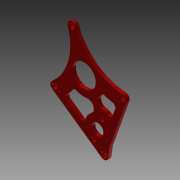
# Autodesk Inventor part: OutlineSketch1
Saved by Autodesk Inventor 2013 (Build 170138000, 138)
## iProperties
Created: 2013-06-03
Part Number: OutlineSketch1
Material: Aluminum 6061
Document SubType Name: Modeling
Designer: mvarma
Density: 2.71 g/cm^3
Author: mvarma
Autodesk Inventor part; units mm, degrees
ref_plane "YZ Plane" through (0, 0, 0) normal (1, 0, 0) x (0, 1, 0)
ref_plane "XZ Plane" through (0, 0, 0) normal (0, 1, 0) x (-1, 0, 0)
ref_plane "XY Plane" through (0, 0, 0) normal (0, 0, 1) x (1, 0, 0)
sketch "Sketch1" plane through (0, 0, 0) normal (0, 0, 1) x (1, 0, 0)
  line L0 (0, 0) -> (304.8, 0) construction
  line L1 (304.8, 0) -> (304.8, 50.8) construction
  line L2 (304.8, 50.8) -> (0, 50.8) construction
  line L3 (0, 50.8) -> (0, 0) construction
  circle A0 centre (152.4, 23.8125) radius 6.35 construction
  circle A1 centre (152.4, 23.8125) radius 34.29 construction
  circle A2 centre (152.4, 23.8125) radius 22.225 construction
  line L4 (152.4, 23.8125) -> (139.52, 61.741) construction
  circle A3 centre (139.52, 61.741) radius 9.525 construction
  circle A4 centre (139.52, 61.741) radius 17.78 construction
  circle A5 centre (91.5619, 85.09) radius 31.75 construction
  circle A6 centre (163.3424, 109.4657) radius 31.75 construction
  circle A7 centre (222.6465, 85.09) radius 31.75 construction
  line L5 (0, 50.8) -> (0, 53.34) construction
  line L6 (0, 53.34) -> (304.8, 53.34) construction
  line L7 (304.8, 53.34) -> (304.8, 50.8) construction
  circle A8 centre (139.52, 61.741) radius 21.59 construction
  circle A9 centre (152.4, 23.8125) radius 46.99 construction
  circle A10 centre (152.4, 23.8125) radius 50.8 construction
  arc A11 (86.3865, 79.4564) -> (92.4363, 92.6899) centre (91.5619, 85.09) ccw construction
  circle A12 centre (163.3424, 109.4657) radius 7.65 construction
  arc A13 (222.2546, 92.73) -> (226.29, 78.3634) centre (222.6465, 85.09) ccw construction
  circle A14 centre (163.3424, 109.4657) radius 9.1 construction
  circle A15 centre (139.52, 61.741) radius 22.9 construction
  line L8 (86.3865, 79.4564) -> (124.0276, 44.8769) construction
  line L9 (170.8782, 108.1486) -> (162.078, 57.7984) construction
  line L10 (92.4363, 92.6899) -> (91.5619, 85.09) construction
  line L11 (91.5619, 85.09) -> (86.3865, 79.4564) construction
  arc A16 (128.9499, 92.8673) -> (131.407, 97.9722) centre (127.6738, 96.6252) ccw
  circle A17 centre (127.6738, 96.6252) radius 7.9375 construction
  line L12 (92.4363, 92.6899) -> (126.7664, 88.7398) construction
  line L13 (133.1953, 90.9229) -> (158.0208, 114.9615) construction
  line L14 (158.0208, 114.9615) -> (163.3424, 109.4657) construction
  line L15 (170.8782, 108.1486) -> (163.3424, 109.4657) construction
  line L16 (139.52, 61.741) -> (127.6738, 96.6252) construction
  line L17 (91.5619, 85.09) -> (163.3424, 109.4657) construction
  line L18 (152.4, 23.8125) -> (91.5619, 85.09) construction
  line L19 (152.4, 23.8125) -> (163.3424, 109.4657) construction
  circle A18 centre (127.6738, 96.6252) radius 9.2075 construction
  circle A19 centre (127.6738, 96.6252) radius 6.1595 construction
  arc A20 (92.4363, 92.6899) -> (86.3865, 79.4564) centre (91.5619, 85.09) ccw construction
  circle A21 centre (163.3424, 109.4657) radius 25.4 construction
  circle A22 centre (222.6465, 85.09) radius 25.4 construction
  line L20 (104.7627, 113.9656) -> (78.361, 56.2144) construction
  circle A23 centre (91.5619, 85.09) radius 25.4 construction
  line L21 (214.0607, 115.6571) -> (231.2324, 54.5229) construction
  line L22 (56.0019, 185.6657) -> (208.4019, 185.6657)
  line L23 (208.4019, 185.6657) -> (208.4019, -4.8343)
  line L24 (208.4019, -4.8343) -> (56.0019, -4.8343)
  line L25 (56.0019, -4.8343) -> (56.0019, 185.6657)
  circle A24 centre (139.52, 61.741) radius 11.1125
  arc A25 (226.1312, 75.4959) -> (221.6192, 95.3086) centre (223.8752, 85.4023) ccw construction
  line L26 (221.4349, 84.7168) -> (229.5152, 60.6363) construction
  line L27 (223.8752, 85.4023) -> (229.5152, 60.6363) construction
  line L28 (221.4349, 84.7168) -> (213.3547, 108.7973) construction
  line L29 (223.8752, 85.4023) -> (218.2352, 110.1682) construction
  arc A26 (212.5972, 111.0549) -> (214.1122, 106.5398) centre (213.3547, 108.7973) ccw construction
  arc A27 (218.764, 107.8464) -> (217.7065, 112.49) centre (218.2352, 110.1682) ccw construction
  arc A28 (218.764, 107.8464) -> (214.1122, 106.5398) centre (229.5152, 60.6363) ccw construction
  arc A29 (217.7065, 112.49) -> (212.5972, 111.0549) centre (229.5152, 60.6363) ccw construction
  line L30 (213.3547, 108.7973) -> (212.5972, 111.0549) construction
  line L31 (218.2352, 110.1682) -> (217.7065, 112.49) construction
  arc A30 (221.6192, 95.3086) -> (218.2029, 94.349) centre (229.5152, 60.6363) ccw construction
  arc A31 (226.1312, 75.4959) -> (224.667, 75.0846) centre (229.5152, 60.6363) ccw construction
  line L32 (104.4015, 107.0791) -> (92.7013, 84.5343) construction
  line L33 (81.0012, 61.9895) -> (90.3961, 85.5882) construction
  arc A32 (100.6718, 111.3992) -> (98.9102, 106.9744) centre (99.791, 109.1868) ccw construction
  arc A33 (103.3046, 104.9655) -> (105.4983, 109.1926) centre (104.4015, 107.0791) ccw construction
  arc A34 (103.3046, 104.9655) -> (98.9102, 106.9744) centre (81.0012, 61.9895) ccw construction
  line L34 (99.791, 109.1868) -> (100.6718, 111.3992) construction
  line L35 (104.4015, 107.0791) -> (105.4983, 109.1926) construction
  arc A35 (105.4983, 109.1926) -> (100.6718, 111.3992) centre (81.0012, 61.9895) ccw construction
  arc A36 (218.2029, 94.349) -> (224.667, 75.0846) centre (221.4349, 84.7168) ccw construction
  arc A37 (88.0213, 75.5164) -> (97.3814, 93.5522) centre (92.7013, 84.5343) ccw construction
  line L36 (90.3961, 85.5882) -> (99.791, 109.1868) construction
  line L37 (92.7013, 84.5343) -> (81.0012, 61.9895) construction
  arc A38 (88.0213, 75.5164) -> (86.6381, 76.1487) centre (81.0012, 61.9895) ccw construction
  arc A39 (97.3814, 93.5522) -> (94.1541, 95.0276) centre (81.0012, 61.9895) ccw construction
  arc A40 (94.1541, 95.0276) -> (86.6381, 76.1487) centre (90.3961, 85.5882) ccw construction
  line L38 (163.3424, 109.4657) -> (140.8985, 121.3583) construction
  line L39 (163.3424, 109.4657) -> (185.7862, 97.5731) construction
  circle A41 centre (139.52, 61.741) radius 26.71 construction
  line L40 (222.2546, 92.73) -> (138.1517, 88.4159) construction
  line L41 (226.29, 78.3634) -> (152.2412, 38.2549) construction
  line L42 (222.6465, 85.09) -> (222.2546, 92.73) construction
  line L43 (222.6465, 85.09) -> (226.29, 78.3634) construction
  line L44 (139.52, 61.741) -> (138.1517, 88.4159) construction
  line L45 (139.52, 61.741) -> (152.2412, 38.2549) construction
  arc A42 (226.29, 78.3634) -> (222.2546, 92.73) centre (222.6465, 85.09) ccw construction
  arc A43 (226.29, 78.3634) -> (225.5574, 78.0155) centre (222.6465, 85.09) ccw construction
  line L46 (139.52, 61.741) -> (222.6465, 85.09) construction
  circle A44 centre (139.52, 61.741) radius 15.875
  arc A45 (108.721, 42.0202) -> (123.8923, 95.4203) centre (76.0203, 80.1659) ccw
  arc A46 (131.407, 97.9722) -> (175.959, 64.8533) centre (178.6686, 115.0239) ccw
  circle A47 centre (152.4, 23.8125) radius 11.176 construction
  line L47 (152.4, 23.8125) -> (158.5256, 5.7742) construction
  circle A48 centre (152.4, 23.8125) radius 5.5065
  line L48 (156.5338, 34.1959) -> (148.2662, 13.4291) construction
  circle A49 centre (156.5338, 34.1959) radius 2.1082
  circle A50 centre (148.2662, 13.4291) radius 2.1082
  arc A51 (166.3874, 21.8643) -> (163.8992, 15.6142) centre (152.4, 23.8125) ccw
  circle A52 centre (111.304, 39.007) radius 9.525 construction
  circle A53 centre (175.745, 60.8903) radius 9.525 construction
  arc A54 (109.2416, 42.3978) -> (109.0199, 35.7614) centre (111.304, 39.007) ccw
  arc A55 (179.4939, 59.5878) -> (175.3161, 64.8358) centre (175.745, 60.8903) ccw
  arc A56 (157.2494, 9.5322) -> (156.2414, 2.5286) centre (158.5256, 5.7742) ccw
  line L49 (152.4, 23.8125) -> (165.1433, 18.7393) construction
  line L50 (166.3874, 21.8643) -> (163.8992, 15.6142)
  arc A57 (163.8992, 15.6142) -> (166.3874, 21.8643) centre (152.4, 23.8125) ccw construction
  line L51 (163.8992, 15.6142) -> (162.4566, 5.2282)
  line L52 (156.2414, 2.5286) -> (109.0199, 35.7614)
  line L53 (166.3874, 21.8643) -> (179.4939, 59.5878)
  arc A58 (175.3161, 64.8358) -> (179.4939, 59.5878) centre (175.745, 60.8903) ccw
  arc A59 (109.0199, 35.7614) -> (109.2416, 42.3978) centre (111.304, 39.007) ccw
  arc A60 (123.8923, 95.4203) -> (128.9499, 92.8673) centre (127.6738, 96.6252) ccw
  arc A61 (131.407, 97.9722) -> (123.8923, 95.4203) centre (127.6738, 96.6252) ccw
  arc A62 (103.6877, 38.2261) -> (108.721, 42.0202) centre (76.0203, 80.1659) ccw
  arc A63 (123.8923, 95.4203) -> (103.6877, 38.2261) centre (76.0203, 80.1659) ccw
  arc A64 (131.202, 98.5513) -> (131.407, 97.9722) centre (178.6686, 115.0239) ccw
  arc A65 (175.959, 64.8533) -> (131.202, 98.5513) centre (178.6686, 115.0239) ccw
  arc A66 (162.4566, 5.2282) -> (157.2494, 9.5322) centre (158.5256, 5.7742) ccw
  arc A67 (156.2414, 2.5286) -> (162.4566, 5.2282) centre (158.5256, 5.7742) ccw
  point P0 (215.7779, 109.5437)
  point P1 (102.1225, 108.1905)
  point P2 (145.0256, 46.8513)
  dimension "d19" = 101.6
  dimension "d127" = 31.75
  dimension "d1" = 50.8
  dimension "d3" = 23.8125
  dimension "d4" = 152.4
  dimension "d7" = 68.58
  dimension "d8" = 44.45
  dimension "d9" = 19.05
  dimension "d10" = 35.56
  dimension "d11" = 40.0558
  dimension "d12" = 63.5
  dimension "d13" = 63.5
  dimension "d14" = 63.5
  dimension "d15" = 2.54
  dimension "d16" = 304.8
  dimension "d17" = 43.18
  dimension "d18" = 93.98
  dimension "d21" = 15.3
  dimension "d22" = 15.3
  dimension "d24" = 18.2
  dimension "d29" = 45.8
  dimension "d30" = 143.991
  dimension "d31" = 7.9375
  dimension "d32" = 15.875
  dimension "d33" = 143.991
  dimension "d35" = 18.415
  dimension "d37" = 12.319
  dimension "d40" = 50.8
  dimension "d41" = 50.8
  dimension "d42" = 18.004
  dimension "d43" = 18.004
  dimension "d44" = 50.8
  dimension "d53" = 152.4
  dimension "d54" = 190.5
  dimension "d55" = 35.56
  dimension "d56" = 76.2
  dimension "d57" = 22.225
  dimension "d67" = 25.4
  dimension "d68" = 25.4
  dimension "d69" = 2.86
  dimension "d70" = 25.4
  dimension "d71" = 25.4
  dimension "d72" = 4.7625
  dimension "d75" = 2.86
  dimension "d80" = 4.7625
  dimension "d82" = 4.7625
  dimension "d83" = 50.8
  dimension "d84" = 50.8
  dimension "d85" = 10.16
  dimension "d97" = 48.4188
  dimension "d99" = 20.32
  dimension "d101" = 25.4
  dimension "d102" = 25.4
  dimension "d103" = 10.16
  dimension "d105" = 18.004
  dimension "d106" = 18.004
  dimension "d107" = 53.42
  dimension "d108" = 154.494
  dimension "d109" = 7.65
  dimension "d111" = 86.3435
  dimension "d112" = 12.753
  dimension "d113" = 12.753
  dimension "d149" = 22.352
  dimension "d152" = 180
  dimension "d163" = 11.013
  dimension "d190" = 12.7
  constraints: 110 end point, 104 point on circle, 66 centre point, 41 coincident, 32 tangent, 17 point on line, 10 collinear, 10 perpendicular, 8 parallel, 4 midpoint, 2 horizontal, 1 equal radius, 1 symmetric about line, 11 other
  measures "d1" distance of L1.end L0.end
  measures "d3" distance from line of L0 A0.centre
  measures "d4" distance from line of L3 A0.centre
  measures "d7" diameter of A1
  measures "d8" diameter of A2
  measures "d9" diameter of A3
  measures "d10" diameter of A4
  measures "d11" distance of L4.start L4.end
  measures "d12" diameter of A5
  measures "d13" diameter of A6
  measures "d14" diameter of A7
  measures "d15" distance of L2.end L5.end
  measures "d16" distance of L0.end L0.start
  measures "d17" diameter of A8
  measures "d18" diameter of A9
  measures "d21" diameter of A11
  measures "d22" diameter of A12
  measures "d24" diameter of A14
  measures "d29" diameter of A15
  measures "d30" angle of L11 L10
  measures "d31" diameter of A16
  measures "d32" diameter of A17
  measures "d33" angle of L15 L14
  measures "d35" diameter of A18
  measures "d37" diameter of A19
  measures "d40" diameter of A21
  measures "d41" diameter of A22
  measures "d42" angle of L10 L20
  measures "d43" angle of L11 L20
  measures "d44" diameter of A23
  measures "d53" distance of L23.end L24.end
  measures "d54" distance of L22.end L23.end
  measures "d55" distance from line of L25 A5.centre
  measures "d56" distance from line of L22 A6.centre
  measures "d57" diameter of A24
  measures "d67" distance of L26.start L26.end
  measures "d68" distance of L27.start L26.end
  measures "d69" angle of L21 L26
  measures "d70" distance of L26.start L28.end
  measures "d71" distance of L27.start L29.end
  measures "d72" diameter of A26
  measures "d75" angle of L20 L32
  measures "d80" diameter of A32
  measures "d82" diameter of A33
  measures "d83" distance of L33.start L36.end
  measures "d84" distance of L32.start L33.start
  measures "d85" radius of A25
  measures "d97" radius of A34
  measures "d99" diameter of A37
  measures "d101" distance of L33.start L33.end
  measures "d102" distance of L32.end L33.start
  measures "d103" radius of A40
  measures "d105" angle of L38 L14
  measures "d106" angle of L39 L15
  measures "d107" diameter of A41
  measures "d108" angle of L42 L43
  measures "d109" radius of A13
  measures "d111" distance of L44.start L42.start
  measures "d112" angle of L21 L42
  measures "d113" angle of L21 L43
  measures "d149" diameter of A47
  measures "d152" angle of L47 L4
  measures "d163" diameter of A48
  measures "d190" diameter of A0
extrude "Extrusion3" add sketch "Sketch1" along normal blind 3.175 contours A60 A61 A16 | A16 A46 A44 A45 A60 | A46 A55 A58 L53 A51 L51 A66 A56 L52 A59 A54 A45 A44 | A44 | A55 A58 | A54 A59 | L50 A51 | A56 A66 A67
hole "Hole3" at (81.0012, 61.9895, 0) at (229.5152, 60.6363, 0) at (185.7862, 97.5731, 0) at (215.7779, 109.5437, 0) at (127.6738, 96.6252, 0) at (111.304, 39.007, 0) at (175.745, 60.8903, 0) at (158.5256, 5.7742, 0) direction (0, 0, 1) diameter 4.9784 end through all clearance for "Socket Head Cap Screw" size "#10" standard "Ansi Unified Screw Threads"
fillet "Fillet3" radius 3.175 2 edges at (166.3874, 21.8643, 1.5875) (163.8992, 15.6142, 1.5875)
sketch "Sketch4" plane through (0, 0, 3.175) normal (0, 0, 1) x (1, 0, 0)
  line L0 (166.4106, 21.931) -> (179.4939, 59.5878) projected
  arc A0 (131.407, 97.9722) -> (175.959, 64.8533) centre (178.6686, 115.0239) ccw projected
  arc A1 (108.721, 42.0202) -> (123.8923, 95.4203) centre (76.0203, 80.1659) ccw projected
  line L1 (109.0199, 35.7614) -> (156.2414, 2.5286) projected
  circle A2 centre (156.5338, 34.1959) radius 2.1082 projected
  circle A3 centre (148.2662, 13.4291) radius 2.1082 projected
  circle A4 centre (152.4, 23.8125) radius 5.5065 projected
  circle A5 centre (139.52, 61.741) radius 11.1125 projected
  circle A6 centre (111.304, 39.007) radius 2.4892 projected
  circle A7 centre (175.745, 60.8903) radius 2.4892 projected
  circle A8 centre (111.304, 39.007) radius 8.8392
  arc A9 (140.8524, 21.1238) -> (146.1133, 33.865) centre (152.4, 23.8125) ccw
  circle A10 centre (148.2662, 13.4291) radius 8.4582
  line L2 (112.6745, 40.9544) -> (120.3925, 35.5227)
  arc A11 (142.1704, 44.4808) -> (153.5844, 51.3906) centre (139.52, 61.741) ccw
  arc A12 (157.4462, 42.6047) -> (164.7065, 36.3748) centre (156.5338, 34.1959) ccw
  circle A13 centre (175.745, 60.8903) radius 8.8392
  arc A14 (119.4607, 93.662) -> (156.1016, 56.2647) centre (178.6686, 115.0239) ccw
  line L3 (160.4123, 24.015) -> (164.7065, 36.3748)
  arc A15 (116.9867, 32.3781) -> (120.3925, 35.5227) centre (76.0203, 80.1659) ccw
  arc A16 (157.4462, 42.6047) -> (153.5844, 51.3906) centre (158.0435, 48.1089) ccw
  arc A17 (142.1704, 44.4808) -> (146.1133, 33.865) centre (143.0479, 38.7666) ccw
  arc A18 (148.5231, 36.9109) -> (142.1704, 44.4808) centre (143.0479, 38.7666) ccw
  arc A19 (146.1133, 33.865) -> (148.5231, 36.9109) centre (143.0479, 38.7666) ccw
  arc A20 (146.1133, 33.865) -> (140.8524, 21.1238) centre (152.4, 23.8125) ccw
  line L4 (140.8524, 21.1238) -> (159.896, 7.7216)
  line L5 (120.3925, 35.5227) -> (140.8524, 21.1238)
  arc A21 (120.3925, 35.5227) -> (129.7021, 47.2998) centre (76.0203, 80.1659) ccw
  arc A22 (129.7021, 47.2998) -> (135.9929, 99.2761) centre (76.0203, 80.1659) ccw
  arc A23 (129.7021, 47.2998) -> (142.1704, 44.4808) centre (139.52, 61.741) ccw
  arc A24 (153.5844, 51.3906) -> (157.4462, 42.6047) centre (158.0435, 48.1089) ccw
  arc A25 (164.7065, 36.3748) -> (157.4462, 42.6047) centre (156.5338, 34.1959) ccw
  line L6 (164.7065, 36.3748) -> (170.3547, 52.6317)
  line L7 (170.3547, 52.6317) -> (173.4956, 61.6718)
  arc A26 (156.1016, 56.2647) -> (170.3547, 52.6317) centre (178.6686, 115.0239) ccw
  arc A27 (170.3547, 52.6317) -> (175.2741, 52.1718) centre (178.6686, 115.0239) ccw
  arc A28 (156.1016, 56.2647) -> (129.7021, 47.2998) centre (139.52, 61.741) ccw
  arc A29 (153.5844, 51.3906) -> (156.1016, 56.2647) centre (139.52, 61.741) ccw
  point P0 (0, 0)
  dimension "d218" = 6.35
  dimension "d219" = 6.35
  dimension "d220" = 6.35
  dimension "d221" = 6.35
  dimension "d222" = 6.35
  dimension "d223" = 6.35
  dimension "d224" = 6.35
  dimension "d225" = 12.7
  dimension "d226" = 6.35
  dimension "d227" = 12.7
  dimension "d228" = 6.35
  constraints: 41 point on circle, 22 centre point, 12 end point, 6 parallel, 5 tangent
  measures "d218" distance between parallel lines of L1 L2
  measures "d219" radial gap between concentric circles of A3 A10
  measures "d220" radial gap between concentric circles of A4 A9
  measures "d221" radial gap between concentric circles of A6 A8
  measures "d222" distance between parallel lines of L0 L3
  measures "d223" radial gap between concentric circles of A2 A12
  measures "d224" radial gap between concentric circles of A7 A13
  measures "d225" radial gap between concentric circles of A0 A14
  measures "d226" radial gap between concentric circles of A11 A5
  measures "d227" radial gap between concentric circles of A1 A15
extrude "Extrusion6" cut sketch "Sketch4" against normal through all contours A26 L6 A25 A16 A29 | A16 A24 | A18 A19 A17 | A17 A20 L5 A21 A23
fillet "Fillet4" radius 3.175 6 edges at (170.3547, 52.6317, 1.5875) (156.1016, 56.2647, 1.5875) (129.7021, 47.2998, 1.5875) (120.3925, 35.5227, 1.5875) (140.8524, 21.1238, 1.5875) (164.7065, 36.3748, 1.5875)
equation "\"d19\" = WheelClearance"
equation "\"d8\" = Gear35tPD"
equation "\"d9\" = Gear15tPD"
equation "\"d10\" = Gear28tPD"
equation "\"d11\" = 0.5 * Gear48tPD + 0.5 * Gear15tPD + MeshingClearance"
equation "\"d12\" = CimOD"
equation "\"d13\" = CimOD"
equation "\"d14\" = CimOD"
equation "\"d17\" = Gear28tPD + ClearanceDiameter"
equation "\"d18\" = WheelOD"
equation "\"Pulley48tPD\" = 45.8"
equation "\"Pulley19tPD\" = 18.2"
equation "\"Pulley16tPD\" = 15.3"
equation "\"Gear15tPD\" = 19.05"
equation "\"Gear35tPD\" = 44.45"
equation "\"Gear48tPD\" = 60.96"
equation "\"Gear28tPD\" = 35.56"
equation "\"BearingLargeOD\" = 28.575"
equation "\"BearingSmallOD\" = 22.225"
equation "\"MeshingClearance\" = 0.0508"
equation "\"CimOD\" = 63.5"
equation "\"WheelOD\" = 93.98"
equation "\"ClearanceDiameter\" = 7.62"
equation "\"WheelClearance\" = 101.6"
equation "\"TensioningBearingID\" = 6.35"
equation "\"TensioningBearingOD\" = 15.875"
equation "\"SpingClipClearance\" = 8.89"
equation "\"Pi\" = 79.79645"
equation "\"Pulley56tPD\" = 53.5"
equation "\"BearingXLargeOD\" = 34.925"
body "Solid3"
